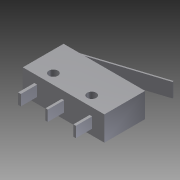
# Autodesk Inventor part: Schalter
Saved by Autodesk Inventor 2012 SP1 (Build 160190100, 190)
## iProperties
Created: 2013-04-29
Part Number: Schalter
Material: Default
Document SubType Name: Modeling
Designer: vogel
Density: 1 g/cm^3
Author: vogel
Autodesk Inventor part; units mm, degrees
ref_plane "YZ Plane" through (0, 0, 0) normal (1, 0, 0) x (0, 1, 0)
ref_plane "XZ Plane" through (0, 0, 0) normal (0, 1, 0) x (-1, 0, 0)
ref_plane "XY Plane" through (0, 0, 0) normal (0, 0, 1) x (1, 0, 0)
sketch "Skizze1" plane through (0, 0, 0) normal (0, 0, 1) x (1, 0, 0)
  line L0 (0, 0) -> (20, 0)
  line L1 (20, 0) -> (20, 10)
  line L2 (20, 10) -> (0, 10)
  line L3 (0, 10) -> (0, 0)
  dimension "d0" = 20
  dimension "d1" = 10
  constraints: 8 end point, 2 parallel, 1 horizontal, 1 perpendicular
  measures "d0" distance of L0.start L0.end
  measures "d1" distance between parallel lines of L2 L0
extrude "Extrusion1" add sketch "Skizze1" along normal blind 6
sketch "Skizze2" plane through (0, 0, 0) normal (0, -1, 0) x (1, 0, 0)
  line L0 (2.8353, 4.0866) -> (3.5144, 4.0866)
  line L1 (3.5144, 4.0866) -> (3.5144, 1.4607)
  line L2 (3.5144, 1.4607) -> (2.8353, 1.4607)
  line L3 (2.8353, 1.4607) -> (2.8353, 4.0866)
  line L4 (9.5586, 4.0866) -> (10.1245, 4.0866)
  line L5 (10.1245, 4.0866) -> (10.1245, 1.4607)
  line L6 (10.1245, 1.4607) -> (9.5586, 1.4607)
  line L7 (9.5586, 1.4607) -> (9.5586, 4.0866)
  line L8 (16.3951, 4.0866) -> (17.0063, 4.0866)
  line L9 (17.0063, 4.0866) -> (17.0063, 1.4607)
  line L10 (17.0063, 1.4607) -> (16.3951, 1.4607)
  line L11 (16.3951, 1.4607) -> (16.3951, 4.0866)
  constraints: 24 end point, 6 parallel, 3 horizontal, 3 perpendicular
extrude "Extrusion2" add sketch "Skizze2" along normal blind 4
sketch "Skizze3" plane through (0, 0, 6) normal (0, 0, 1) x (1, 0, 0)
  line L0 (0, 0) -> (0, 10) projected
  line L1 (20, 0) -> (0, 0) projected
  line L2 (20, 10) -> (20, 0) projected
  line L3 (0, 2.5) -> (20, 2.5)
  point P0 (5, 2.5)
  point P1 (14.4, 2.5)
  dimension "d6" = 2.5
  dimension "d7" = 5
  dimension "d8" = 9.4
  dimension "d9" = 5.6
  constraints: 4 point on line, 2 end point, 1 perpendicular
  measures "d6" distance between parallel lines of L3 L1
  measures "d7" distance from line of L0 point (5, 2.5)
  measures "d8" distance of point (14.4, 2.5) point (5, 2.5)
  measures "d9" distance from line of L2 point (14.4, 2.5)
hole "Bohrung1" at (5, 2.5, 6) at (14.4, 2.5, 6) direction (0, 0, -1) diameter 2.2 end through all
sketch "Skizze4" plane through (0, 10, 0) normal (0, 1, 0) x (1, 0, 0)
  line L0 (5.2978, -1.9699) -> (6.366, -1.9699)
  line L1 (6.366, -1.9699) -> (6.366, -4.0301)
  line L2 (6.366, -4.0301) -> (5.2978, -4.0301)
  line L3 (5.2978, -4.0301) -> (5.2978, -1.9699)
  constraints: 8 end point, 2 parallel, 1 horizontal, 1 perpendicular
extrude "Extrusion3" add sketch "Skizze4" along normal blind 1.5
ref_plane "Arbeitsebene1" through (0, 0, 3) normal (0, 0, 1) x (1, 0, 0)
sketch "Skizze5" plane through (0, 0, 3) normal (0, 0, 1) x (1, 0, 0)
  circle A0 centre (14.4, 2.5) radius 1.1 projected
  circle A1 centre (5, 2.5) radius 1.1 projected
  line L0 (0, 0) -> (0, 10) projected
  line L1 (20, 0) -> (0, 0) projected
  line L2 (20, 10) -> (20, 0) projected
  line L3 (0, 10) -> (20, 10) projected
  line L4 (0, 10) -> (20.2246, 16.5)
  line L5 (20.2246, 16.5) -> (20.1156, 16.839)
  line L6 (20.1156, 16.839) -> (-0.1089, 10.339)
  line L7 (-0.1089, 10.339) -> (0, 10)
  dimension "d20" = 14
  constraints: 8 end point, 2 parallel, 1 perpendicular
  measures "d20" vertical distance of L4.end A0.centre
extrude "Extrusion4" add sketch "Skizze5" along normal mid plane 3.5 contours L7 L6 L5 L4
